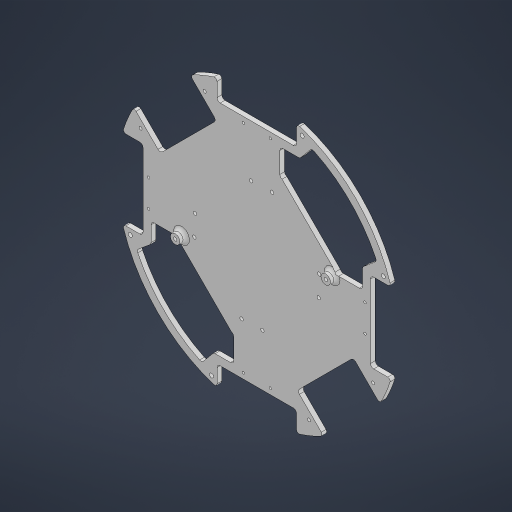
# Autodesk Inventor part: SecondPlate
Saved by Autodesk Inventor 2024.2 (Build 282272000, 272)
## iProperties
Created: 2023-12-22
Part Number: SecondPlate
Material: 一般
Document SubType Name: Modeling
Designer: Hanaoka
Density: 1 g/cm^3
Appearance: 既定
Author: Hanaoka
Autodesk Inventor part; units mm, degrees
(part 1 of 2)
ref_plane "YZ Plane" through (0, 0, 0) normal (1, 0, 0) x (0, 1, 0)
ref_plane "XZ Plane" through (0, 0, 0) normal (0, 1, 0) x (-1, 0, 0)
ref_plane "XY Plane" through (0, 0, 0) normal (0, 0, 1) x (1, 0, 0)
sketch "スケッチ1" plane through (0, 0, 0) normal (0, 0, 1) x (1, 0, 0)
  arc A0 (4.2199, -1.5405) -> (-52.5892, 55.2686) centre (-79.5487, -28.5) ccw projected
  arc A1 (2.792, -3.5) -> (4.2199, -1.5405) centre (2.792, -2) ccw projected
  line L0 (-6.0487, -3.5) -> (2.792, -3.5) projected
  circle A2 centre (0, 0) radius 2.5 projected
  circle A3 centre (0, 0) radius 1.3 projected
  arc A4 (-6.0487, -3.5) -> (-8.0487, -5.5) centre (-6.0487, -5.5) ccw projected
  line L1 (-8.0487, -51.5) -> (-8.0487, -5.5) projected
  arc A5 (-8.0487, -51.5) -> (-6.0487, -53.5) centre (-6.0487, -51.5) ccw projected
  line L2 (2.792, -53.5) -> (-6.0487, -53.5) projected
  arc A6 (4.2199, -55.4595) -> (2.792, -53.5) centre (2.792, -55) ccw projected
  arc A7 (-1.2521, -68.6701) -> (4.2199, -55.4595) centre (-79.5487, -28.5) ccw projected
  arc A8 (-3.6474, -69.046) -> (-1.2521, -68.6701) centre (-2.5867, -67.9854) ccw projected
  line L3 (-9.6341, -63.0593) -> (-3.6474, -69.046) projected
  arc A9 (-9.6341, -63.0593) -> (-13.8768, -63.0593) centre (-11.7555, -65.1806) ccw projected
  line L4 (-15.892, -65.0745) -> (-13.8768, -63.0593) projected
  line L5 (-39.4387, -88.6212) -> (-19.4276, -68.61) projected
  line L6 (-44.9895, -94.172) -> (-42.9742, -92.1567) projected
  arc A10 (-44.9895, -94.172) -> (-44.9895, -98.4146) centre (-42.8682, -96.2933) ccw projected
  line L7 (-39.0027, -104.4014) -> (-44.9895, -98.4146) projected
  arc A11 (-39.3786, -106.7966) -> (-39.0027, -104.4014) centre (-40.0634, -105.462) ccw projected
  arc A12 (-52.5892, -112.2686) -> (-39.3786, -106.7966) centre (-79.5487, -28.5) ccw projected
  arc A13 (-54.5487, -110.8408) -> (-52.5892, -112.2686) centre (-53.0487, -110.8408) ccw projected
  line L8 (-54.5487, -102) -> (-54.5487, -110.8408) projected
  arc A14 (-54.5487, -102) -> (-56.5487, -100) centre (-56.5487, -102) ccw projected
  line L9 (-102.5487, -100) -> (-56.5487, -100) projected
  arc A15 (-102.5487, -100) -> (-104.5487, -102) centre (-102.5487, -102) ccw projected
  line L10 (-104.5487, -110.8408) -> (-104.5487, -102) projected
  arc A16 (-106.5083, -112.2686) -> (-104.5487, -110.8408) centre (-106.0487, -110.8408) ccw projected
  arc A17 (-163.3174, -55.4595) -> (-106.5083, -112.2686) centre (-79.5487, -28.5) ccw projected
  circle A18 centre (-108.0487, -108.0487) radius 2.5 projected
  circle A19 centre (-108.0487, -108.0487) radius 1.3 projected
  arc A20 (-161.8895, -53.5) -> (-163.3174, -55.4595) centre (-161.8895, -55) ccw projected
  line L11 (-153.0487, -53.5) -> (-161.8895, -53.5) projected
  circle A21 centre (-159.0975, -57) radius 1.3 projected
  circle A22 centre (-159.0975, -57) radius 2.5 projected
  arc A23 (-153.0487, -53.5) -> (-151.0487, -51.5) centre (-153.0487, -51.5) ccw projected
  line L12 (-151.0487, -5.5) -> (-151.0487, -51.5) projected
  line L13 (-161.8895, -3.5) -> (-153.0487, -3.5) projected
  arc A24 (-151.0487, -5.5) -> (-153.0487, -3.5) centre (-153.0487, -5.5) ccw projected
  arc A25 (-163.3174, -1.5405) -> (-161.8895, -3.5) centre (-161.8895, -2) ccw projected
  arc A26 (-157.8454, 11.6701) -> (-163.3174, -1.5405) centre (-79.5487, -28.5) ccw projected
  arc A27 (-155.4501, 12.046) -> (-157.8454, 11.6701) centre (-156.5108, 10.9854) ccw projected
  line L14 (-149.4633, 6.0593) -> (-155.4501, 12.046) projected
  arc A28 (-149.4633, 6.0593) -> (-145.2207, 6.0593) centre (-147.342, 8.1806) ccw projected
  line L15 (-143.2054, 8.0745) -> (-145.2207, 6.0593) projected
  line L16 (-119.6588, 31.6212) -> (-139.6699, 11.61) projected
  line L17 (-114.108, 37.172) -> (-116.1232, 35.1567) projected
  arc A29 (-114.108, 37.172) -> (-114.108, 41.4146) centre (-116.2293, 39.2933) ccw projected
  line L18 (-120.0948, 47.4014) -> (-114.108, 41.4146) projected
  arc A30 (-119.7188, 49.7966) -> (-120.0948, 47.4014) centre (-119.0341, 48.462) ccw projected
  arc A31 (-106.5083, 55.2686) -> (-119.7188, 49.7966) centre (-79.5487, -28.5) ccw projected
  arc A32 (-104.5487, 53.8408) -> (-106.5083, 55.2686) centre (-106.0487, 53.8408) ccw projected
  line L19 (-104.5487, 45) -> (-104.5487, 53.8408) projected
  arc A33 (-104.5487, 45) -> (-102.5487, 43) centre (-102.5487, 45) ccw projected
  line L20 (-56.5487, 43) -> (-102.5487, 43) projected
  arc A34 (-52.5892, 55.2686) -> (-54.5487, 53.8408) centre (-53.0487, 53.8408) ccw projected
  line L21 (-54.5487, 53.8408) -> (-54.5487, 45) projected
  arc A35 (-56.5487, 43) -> (-54.5487, 45) centre (-56.5487, 45) ccw projected
  circle A36 centre (-51.0487, 51.0487) radius 2.5 projected
  circle A37 centre (-51.0487, 51.0487) radius 1.3 projected
  circle A38 centre (-11.5487, -37) radius 0.8 projected
  circle A39 centre (-11.5487, -20) radius 0.8 projected
  line L22 (-9.5487, -39.5) -> (-9.5487, -17.5) projected
  line L23 (-9.5487, -17.5) -> (-13.5487, -17.5) projected
  line L24 (-13.5487, -39.5) -> (-13.5487, -17.5) projected
  line L25 (-9.5487, -39.5) -> (-13.5487, -39.5) projected
  circle A40 centre (-71.0487, 39.5) radius 0.8 projected
  circle A41 centre (-88.0487, 39.5) radius 0.8 projected
  line L26 (-68.5487, 41.5) -> (-90.5487, 41.5) projected
  line L27 (-90.5487, 41.5) -> (-90.5487, 37.5) projected
  line L28 (-68.5487, 37.5) -> (-90.5487, 37.5) projected
  line L29 (-68.5487, 41.5) -> (-68.5487, 37.5) projected
  circle A42 centre (-147.5487, -20) radius 0.8 projected
  circle A43 centre (-147.5487, -37) radius 0.8 projected
  line L30 (-149.5487, -17.5) -> (-149.5487, -39.5) projected
  line L31 (-149.5487, -39.5) -> (-145.5487, -39.5) projected
  line L32 (-145.5487, -17.5) -> (-145.5487, -39.5) projected
  line L33 (-149.5487, -17.5) -> (-145.5487, -17.5) projected
  circle A44 centre (-88.0487, -96.5) radius 0.8 projected
  circle A45 centre (-71.0487, -96.5) radius 0.8 projected
  line L34 (-90.5487, -98.5) -> (-68.5487, -98.5) projected
  line L35 (-68.5487, -98.5) -> (-68.5487, -94.5) projected
  line L36 (-90.5487, -94.5) -> (-68.5487, -94.5) projected
  line L37 (-90.5487, -98.5) -> (-90.5487, -94.5) projected
  line L38 (-116.1232, 35.1567) -> (-119.6588, 31.6212)
  line L39 (-139.6699, 11.61) -> (-143.2054, 8.0745)
  line L40 (-15.892, -65.0745) -> (-19.4276, -68.61)
  line L41 (-42.9742, -92.1567) -> (-42.4775, -91.66)
  line L42 (-42.4775, -91.66) -> (-39.4387, -88.6212)
  line L43 (-49.5487, 45.911) -> (-49.5487, 38)
  line L44 (-51.5487, 36) -> (-72.0251, 36)
  line L45 (-73.4393, 35.4142) -> (-143.4629, -34.6094)
  line L46 (-5.1377, 1.5) -> (-13.0487, 1.5)
  line L47 (-15.0487, -0.5) -> (-15.0487, -20.9764)
  line L48 (-15.6345, -22.3906) -> (-85.6581, -92.4142)
  arc A46 (-3.3004, 4.2901) -> (-46.7586, 47.7483) centre (-79.5487, -28.5) ccw
  arc A47 (-5.1377, 1.5) -> (-3.3004, 4.2901) centre (-5.1377, 3.5) ccw
  arc A48 (-46.7586, 47.7483) -> (-49.5487, 45.911) centre (-47.5487, 45.911) ccw
  arc A49 (-51.5487, 36) -> (-49.5487, 38) centre (-51.5487, 38) ccw
  arc A50 (-13.0487, 1.5) -> (-15.0487, -0.5) centre (-13.0487, -0.5) ccw
  arc A51 (-15.6345, -22.3906) -> (-15.0487, -20.9764) centre (-17.0487, -20.9764) ccw
  arc A52 (-72.0251, 36) -> (-73.4393, 35.4142) centre (-72.0251, 34) ccw
  line L49 (-129.6643, 21.6156) -> (-29.4331, -78.6156) construction
  line L50 (-153.9597, -58.5) -> (-146.0487, -58.5)
  line L51 (-144.0487, -56.5) -> (-144.0487, -36.0236)
  line L52 (-109.5487, -102.911) -> (-109.5487, -95)
  line L53 (-107.5487, -93) -> (-87.0724, -93)
  arc A53 (-155.7971, -61.2901) -> (-112.3389, -104.7483) centre (-79.5487, -28.5) ccw
  arc A54 (-112.3389, -104.7483) -> (-109.5487, -102.911) centre (-111.5487, -102.911) ccw
  arc A55 (-153.9597, -58.5) -> (-155.7971, -61.2901) centre (-153.9597, -60.5) ccw
  arc A56 (-146.0487, -58.5) -> (-144.0487, -56.5) centre (-146.0487, -56.5) ccw
  arc A57 (-107.5487, -93) -> (-109.5487, -95) centre (-107.5487, -95) ccw
  arc A58 (-87.0724, -93) -> (-85.6581, -92.4142) centre (-87.0724, -91) ccw
  arc A59 (-143.4629, -34.6094) -> (-144.0487, -36.0236) centre (-142.0487, -36.0236) ccw
  line L54 (-9.6341, -63.0593) -> (-36.5042, -36.1892)
  line L55 (-39.3326, -36.1892) -> (-71.8595, -68.7161)
  line L56 (-71.8595, -71.5445) -> (-44.9895, -98.4146)
  arc A60 (-36.5042, -36.1892) -> (-39.3326, -36.1892) centre (-37.9184, -37.6034) ccw
  arc A61 (-71.8595, -68.7161) -> (-71.8595, -71.5445) centre (-70.4453, -70.1303) ccw
  line L57 (-114.108, 41.4146) -> (-87.2379, 14.5445)
  line L58 (-87.2379, 11.7161) -> (-119.7648, -20.8108)
  line L59 (-122.5933, -20.8108) -> (-149.4633, 6.0593)
  arc A62 (-87.2379, 11.7161) -> (-87.2379, 14.5445) centre (-88.6521, 13.1303) ccw
  arc A63 (-122.5933, -20.8108) -> (-119.7648, -20.8108) centre (-121.179, -19.3966) ccw
  arc A64 (4.2199, -55.4595) -> (4.2199, -55.4595) centre (-79.5487, -28.5) ccw
  arc A65 (-52.5892, -112.2686) -> (-52.5892, -112.2686) centre (-79.5487, -28.5) ccw
  arc A66 (-54.5487, -102) -> (-56.5487, -100) centre (-56.5487, -102) ccw
  point P0 (0, 0)
  point P1 (-49.5487, 48.8886)
  point P2 (-2.1601, 1.5)
  point P3 (-2.1601, 1.5)
  point P4 (-49.5487, 48.8886)
  point P5 (-73.2737, -70.1303)
  point P6 (-52.5892, -112.2686)
  dimension "d2" = 5
  dimension "d3" = 2
  dimension "d4" = 5
  dimension "d5" = 5
  dimension "d6" = 1.5
  dimension "d7" = 1.5
  dimension "d8" = 30
  dimension "d9" = 30
  dimension "d12" = 40
  dimension "d13" = 2
  constraints: 47 point on circle, 44 end point, 21 centre point, 20 tangent, 19 symmetric about line, 11 parallel, 8 equal radius, 8 point on line, 4 collinear, 3 coincident, 2 midpoint, 1 perpendicular, 8 other
  measures "d2" radial gap between concentric circles of A0 A46
  measures "d3" radius of A47
  measures "d4" distance between parallel lines of L0 L46
  measures "d5" distance between parallel lines of L21 L43
  measures "d6" distance between parallel lines of L44 L28
  measures "d7" distance between parallel lines of L47 L24
  measures "d8" distance between parallel lines of L16 L45
  measures "d9" distance between parallel lines of L5 L48
  measures "d12" distance of point (-73.274, -70.13) L7.end
  measures "d13" radius of A60
extrude "押し出し1" add sketch "スケッチ1" along normal blind 1 contours A1 L0 A4 L1 A5 L2 A6 A7 A8 L3 L54 L48 A51 L47 A50 L46 A47 A46 A48 L43 A49 L44 A52 L45 L57 L18 A30 A31 A32 L19 A33 L20 A35 L21 A34 A0 | A27 L14 L59 L45 A59 L51 A56 L50 A55 A53 A54 L52 A57 L53 A58 L48 L56 L7 A11 A12 A13 L8 A14 L9 A15 L10 A16 A17 A20 L11 A23 L12 A24 L13 A25 A26 | L57 A62 L58 A63 L59 L45 | L45 A52 L44 A49 L43 A48 A46 A47 L46 A50 L47 A51 L48 L54 A60 L55 A61 L56 A58 L53 A57 L52 A54 A53 A55 L50 A56 L51 A59 L59 A63 L58 A62 L57 | L48 L56 A61 L55 A60 L54 | A2 | A18 | A22 | A36 | L25 L24 L23 L22 | L29 L28 L27 L26 | L33 L32 L31 L30 | L37 L36 L35 L34
sketch "スケッチ2" plane through (0, 0, 0) normal (0, 0, -1) x (-1, 0, 0)
  arc A0 (-4.2199, -1.5405) -> (-2.792, -3.5) centre (-2.792, -2) ccw projected
  line L0 (6.0487, -3.5) -> (-2.792, -3.5) projected
  arc A1 (8.0487, -5.5) -> (6.0487, -3.5) centre (6.0487, -5.5) ccw projected
  line L1 (8.0487, -51.5) -> (8.0487, -5.5) projected
  arc A2 (6.0487, -53.5) -> (8.0487, -51.5) centre (6.0487, -51.5) ccw projected
  line L2 (-2.792, -53.5) -> (6.0487, -53.5) projected
  arc A3 (-2.792, -53.5) -> (-4.2199, -55.4595) centre (-2.792, -55) ccw projected
  arc A4 (-4.2199, -55.4595) -> (1.2521, -68.6701) centre (79.5487, -28.5) ccw projected
  arc A5 (1.2521, -68.6701) -> (3.6474, -69.046) centre (2.5867, -67.9854) ccw projected
  line L3 (32.9687, -39.7247) -> (3.6474, -69.046) projected
  line L4 (39.0027, -104.4014) -> (68.324, -75.0801) projected
  arc A6 (39.0027, -104.4014) -> (39.3786, -106.7966) centre (40.0634, -105.462) ccw projected
  arc A7 (39.3786, -106.7966) -> (52.5892, -112.2686) centre (79.5487, -28.5) ccw projected
  arc A8 (52.5892, -112.2686) -> (54.5487, -110.8408) centre (53.0487, -110.8408) ccw projected
  line L5 (54.5487, -102) -> (54.5487, -110.8408) projected
  arc A9 (56.5487, -100) -> (54.5487, -102) centre (56.5487, -102) ccw projected
  line L6 (102.5487, -100) -> (56.5487, -100) projected
  arc A10 (104.5487, -102) -> (102.5487, -100) centre (102.5487, -102) ccw projected
  line L7 (104.5487, -110.8408) -> (104.5487, -102) projected
  arc A11 (104.5487, -110.8408) -> (106.5083, -112.2686) centre (106.0487, -110.8408) ccw projected
  arc A12 (106.5083, -112.2686) -> (163.3174, -55.4595) centre (79.5487, -28.5) ccw projected
  arc A13 (163.3174, -55.4595) -> (161.8895, -53.5) centre (161.8895, -55) ccw projected
  line L8 (153.0487, -53.5) -> (161.8895, -53.5) projected
  arc A14 (151.0487, -51.5) -> (153.0487, -53.5) centre (153.0487, -51.5) ccw projected
  line L9 (151.0487, -5.5) -> (151.0487, -51.5) projected
  arc A15 (153.0487, -3.5) -> (151.0487, -5.5) centre (153.0487, -5.5) ccw projected
  line L10 (161.8895, -3.5) -> (153.0487, -3.5) projected
  arc A16 (161.8895, -3.5) -> (163.3174, -1.5405) centre (161.8895, -2) ccw projected
  arc A17 (163.3174, -1.5405) -> (157.8454, 11.6701) centre (79.5487, -28.5) ccw projected
  arc A18 (157.8454, 11.6701) -> (155.4501, 12.046) centre (156.5108, 10.9854) ccw projected
  line L11 (126.1288, -17.2753) -> (155.4501, 12.046) projected
  line L12 (120.0948, 47.4014) -> (90.7735, 18.0801) projected
  arc A19 (120.0948, 47.4014) -> (119.7188, 49.7966) centre (119.0341, 48.462) ccw projected
  arc A20 (119.7188, 49.7966) -> (106.5083, 55.2686) centre (79.5487, -28.5) ccw projected
  arc A21 (106.5083, 55.2686) -> (104.5487, 53.8408) centre (106.0487, 53.8408) ccw projected
  line L13 (104.5487, 45) -> (104.5487, 53.8408) projected
  arc A22 (102.5487, 43) -> (104.5487, 45) centre (102.5487, 45) ccw projected
  line L14 (56.5487, 43) -> (102.5487, 43) projected
  arc A23 (54.5487, 45) -> (56.5487, 43) centre (56.5487, 45) ccw projected
  line L15 (54.5487, 53.8408) -> (54.5487, 45) projected
  arc A24 (54.5487, 53.8408) -> (52.5892, 55.2686) centre (53.0487, 53.8408) ccw projected
  arc A25 (52.5892, 55.2686) -> (-4.2199, -1.5405) centre (79.5487, -28.5) ccw projected
  line L16 (68.5487, 37.5) -> (90.5487, 37.5) projected
  line L17 (68.5487, 41.5) -> (90.5487, 41.5) projected
  line L18 (90.5487, 41.5) -> (90.5487, 37.5) projected
  line L19 (68.5487, 41.5) -> (68.5487, 37.5) projected
  line L20 (149.5487, -17.5) -> (149.5487, -39.5) projected
  line L21 (149.5487, -17.5) -> (145.5487, -17.5) projected
  line L22 (145.5487, -17.5) -> (145.5487, -39.5) projected
  line L23 (149.5487, -39.5) -> (145.5487, -39.5) projected
  line L24 (90.5487, -98.5) -> (68.5487, -98.5) projected
  line L25 (90.5487, -94.5) -> (68.5487, -94.5) projected
  line L26 (90.5487, -98.5) -> (90.5487, -94.5) projected
  line L27 (68.5487, -98.5) -> (68.5487, -94.5) projected
  line L28 (13.5487, -39.5) -> (13.5487, -17.5) projected
  line L29 (9.5487, -17.5) -> (13.5487, -17.5) projected
  line L30 (9.5487, -39.5) -> (9.5487, -17.5) projected
  line L31 (9.5487, -39.5) -> (13.5487, -39.5) projected
  circle A26 centre (51.0487, 51.0487) radius 2.5
  circle A27 centre (0, 0) radius 2.5
  circle A28 centre (159.0975, -57) radius 2.5
  circle A29 centre (108.0487, -108.0487) radius 2.5
  line L32 (17.3233, 33.7254) -> (141.7741, -90.7254) construction
  circle A30 centre (118.7932, -38.0459) radius 1.1
  circle A31 centre (89.0947, -67.7444) radius 1.1
  line L33 (118.7932, -38.0459) -> (89.0947, -67.7444) construction
  line L34 (114.108, 6.0593) -> (44.9895, -63.0593) construction
  circle A32 centre (70.0028, 10.7444) radius 1.1
  circle A33 centre (40.3043, -18.9541) radius 1.1
  line L35 (70.0028, 10.7444) -> (40.3043, -18.9541) construction
  line L36 (149.5487, -17.5) -> (149.1952, -17.8536) construction
  arc A34 (149.5487, -18.2071) -> (148.8416, -17.5) centre (149.1952, -17.8536) ccw
  line L37 (149.1952, -17.5) -> (149.1952, -17.8536) construction
  line L38 (149.1952, -17.8536) -> (149.5487, -17.8536) construction
  line L39 (145.5487, -17.5) -> (145.9023, -17.8536) construction
  line L40 (149.5487, -39.5) -> (149.1952, -39.1464) construction
  line L41 (145.5487, -39.5) -> (145.9023, -39.1464) construction
  line L42 (145.9023, -17.8536) -> (145.9023, -17.5) construction
  line L43 (145.9023, -17.8536) -> (145.5487, -17.8536) construction
  line L44 (149.1952, -39.1464) -> (149.5487, -39.1464) construction
  line L45 (145.9023, -39.1464) -> (145.5487, -39.1464) construction
  line L46 (145.9023, -39.1464) -> (145.9023, -39.5) construction
  line L47 (149.1952, -39.1464) -> (149.1952, -39.5) construction
  arc A35 (146.2558, -17.5) -> (145.5487, -18.2071) centre (145.9023, -17.8536) ccw
  arc A36 (148.8416, -39.5) -> (149.5487, -38.7929) centre (149.1952, -39.1464) ccw
  arc A37 (145.5487, -38.7929) -> (146.2558, -39.5) centre (145.9023, -39.1464) ccw
  arc A38 (69.2558, 41.5) -> (68.5487, 40.7929) centre (68.9023, 41.1464) ccw
  arc A39 (68.5487, 38.2071) -> (69.2558, 37.5) centre (68.9023, 37.8536) ccw
  arc A40 (90.5487, 40.7929) -> (89.8416, 41.5) centre (90.1952, 41.1464) ccw
  arc A41 (89.8416, 37.5) -> (90.5487, 38.2071) centre (90.1952, 37.8536) ccw
  arc A42 (9.5487, -38.7929) -> (10.2558, -39.5) centre (9.9023, -39.1464) ccw
  arc A43 (12.8416, -39.5) -> (13.5487, -38.7929) centre (13.1952, -39.1464) ccw
  arc A44 (10.2558, -17.5) -> (9.5487, -18.2071) centre (9.9023, -17.8536) ccw
  arc A45 (13.5487, -18.2071) -> (12.8416, -17.5) centre (13.1952, -17.8536) ccw
  arc A46 (89.8416, -98.5) -> (90.5487, -97.7929) centre (90.1952, -98.1464) ccw
  arc A47 (90.5487, -95.2071) -> (89.8416, -94.5) centre (90.1952, -94.8536) ccw
  arc A48 (68.5487, -97.7929) -> (69.2558, -98.5) centre (68.9023, -98.1464) ccw
  arc A49 (69.2558, -94.5) -> (68.5487, -95.2071) centre (68.9023, -94.8536) ccw
  line L48 (68.324, -75.0801) -> (32.9687, -39.7247) projected
  line L49 (90.7735, 18.0801) -> (126.1288, -17.2753) projected
  circle A50 centre (88.0487, 39.5) radius 0.8 projected
  circle A51 centre (71.0487, 39.5) radius 0.8 projected
  circle A52 centre (147.5487, -20) radius 0.8 projected
  circle A53 centre (147.5487, -37) radius 0.8 projected
  circle A54 centre (88.0487, -96.5) radius 0.8 projected
  circle A55 centre (71.0487, -96.5) radius 0.8 projected
  circle A56 centre (11.5487, -20) radius 0.8 projected
  circle A57 centre (11.5487, -37) radius 0.8 projected
  circle A58 centre (0, 0) radius 1.3 projected
  circle A59 centre (51.0487, 51.0487) radius 1.3 projected
  circle A60 centre (159.0975, -57) radius 1.3 projected
  circle A61 centre (108.0487, -108.0487) radius 1.3 projected
  point P0 (0, 0)
  point P1 (103.9439, -52.8952)
  point P2 (79.5487, -28.5)
  point P3 (68.5487, 41.5)
  point P4 (9.5487, -39.5)
  point P5 (90.5487, -98.5)
  point P6 (69.2558, 37.5)
  point P7 (13.5487, -38.7929)
  point P8 (68.5487, -95.2071)
  point P9 (69.2558, -94.5)
  point P10 (89.8416, -94.5)
  point P11 (90.5487, -97.7929)
  point P12 (89.8416, -98.5)
  point P13 (69.2558, -98.5)
  dimension "d16" = 5
  dimension "d17" = 2.2
  dimension "d18" = 42
  dimension "d19" = 34.5
  dimension "d20" = 34.5
  dimension "d61" = 0.5
  dimension "d65" = 360
  constraints: 38 point on circle, 32 end point, 24 centre point, 17 point on line, 8 equal length, 8 equal radius, 4 coincident, 4 perpendicular, 3 parallel, 2 midpoint, 1 vertical, 71 other
  measures "d16" diameter of A26
  measures "d17" diameter of A31
  measures "d18" distance of L33.start L33.end
  measures "d19" distance of point (103.944, -52.895) point (79.549, -28.5)
  measures "d20" distance between parallel lines of L34 L35
  measures "d61" distance of L20.start L36.end
extrude "押し出し2" add sketch "スケッチ2" along normal blind 2 contours A25 A24 L15 A23 L14 A22 L13 A21 A20 A19 L12 L49 L11 A18 A17 A16 L10 A15 L9 A14 L8 A13 A12 A11 L7 A10 L6 A9 L5 A8 A7 A6 L4 L48 L3 A5 A4 A3 L2 A2 L1 A1 L0 A0 | L19 L17 L18 L16 | A39 L19 | L16 A39 | L16 A41 | A38 L19 | L18 A41 | A38 L17 | L18 A40 | A40 L17 | A34 L20 | L20 L23 L22 L21 | L21 A34 | A36 L20 | L21 A35 | A36 L23 | L22 A35 | A37 L23 | L22 A37 | A46 L24 | L24 L27 L25 L26 | L26 A46 | A48 L24 | L26 A47 | A48 L27 | L25 A47 | A49 L27 | L25 A49 | L31 L30 L29 L28 | A43 L31 | L28 A43 | L28 A45 | A42 L31 | L29 A45 | A42 L30 | L29 A44 | A44 L30 | A26 | A27 | A28 | A29 | A30 | A31 | A32 | A33
extrude "押し出し3" cut sketch "スケッチ2" along normal mid plane 5 contours A30 | A31 | A32 | A33
sketch "スケッチ3" plane through (0, 0, 1) normal (0, 0, 1) x (1, 0, 0)
  circle A0 centre (-40.6579, -32.0355) radius 1.1
  circle A1 centre (-76.0132, -67.3909) radius 1.1
  circle A2 centre (-83.0843, 10.3909) radius 1.1
  circle A3 centre (-118.4396, -24.9645) radius 1.1
  line L0 (-83.0843, 10.3909) -> (-40.6579, -32.0355) construction
  line L1 (-40.6579, -32.0355) -> (-76.0132, -67.3909) construction
  line L2 (-76.0132, -67.3909) -> (-118.4396, -24.9645) construction
  line L3 (-118.4396, -24.9645) -> (-83.0843, 10.3909) construction
  line L4 (-17.3233, 33.7254) -> (-141.7741, -90.7254) construction
  arc A4 (4.2199, -1.5405) -> (-52.5892, 55.2686) centre (-79.5487, -28.5) ccw projected
  arc A5 (-163.3174, -55.4595) -> (-106.5083, -112.2686) centre (-79.5487, -28.5) ccw projected
  line L5 (-97.8445, 22.3227) -> (-130.3714, -10.2042) projected
  line L6 (-114.108, 6.0593) -> (-44.9895, -63.0593) construction
  line L7 (-61.2529, -79.3227) -> (-28.726, -46.7958) projected
  circle A6 centre (-40.6579, -32.0355) radius 2.5
  circle A7 centre (-76.0132, -67.3909) radius 2.5
  circle A8 centre (-118.4396, -24.9645) radius 2.5
  circle A9 centre (-83.0843, 10.3909) radius 2.5
  point P0 (0, 0)
  point P1 (-58.3355, -49.7132)
  point P2 (-97.2264, -46.1777)
  dimension "d23" = 2.2
  dimension "d24" = 50
  dimension "d25" = 60
  dimension "d26" = 5
  constraints: 12 end point, 8 centre point, 6 equal radius, 4 coincident, 4 midpoint, 4 parallel, 2 point on circle, 2 point on line
  measures "d23" diameter of A1
  measures "d24" distance of L0.end L1.end
  measures "d25" distance of L0.start L0.end
  measures "d26" diameter of A7
extrude "押し出し4" cut sketch "スケッチ3" against normal up to surface (3 mm away) contours A0 | A1 | A2 | A3
sketch "スケッチ5" plane through (0, 0, 1) normal (0, 0, 1) x (1, 0, 0)
  arc A0 (-25.87, 37.9067) -> (-25.9576, 39.3987) centre (-26.5771, 38.6138) ccw projected
  arc A1 (-25.9576, 39.3987) -> (-45.1385, 50.8611) centre (-79.5487, -28.5) ccw projected
  arc A2 (-45.1385, 50.8611) -> (-47.4757, 50.3004) centre (-45.9341, 49.0262) ccw projected
  line L0 (-47.4757, 50.3004) -> (-53.7364, 42.7258) projected
  arc A3 (-55.278, 42) -> (-53.7364, 42.7258) centre (-55.278, 44) ccw projected
  line L1 (-55.278, 42) -> (-63.0487, 42) projected
  arc A4 (-63.0487, 42) -> (-65.0487, 40) centre (-63.0487, 40) ccw projected
  line L2 (-65.0487, 40) -> (-65.0487, 27.1035) projected
  arc A5 (-65.0487, 27.1035) -> (-63.6177, 25.1861) centre (-63.0487, 27.1035) ccw projected
  arc A6 (-25.8626, -12.569) -> (-63.6177, 25.1861) centre (-79.5487, -28.5) ccw projected
  arc A7 (-25.8626, -12.569) -> (-23.9452, -14) centre (-23.9452, -12) ccw projected
  line L3 (-23.9452, -14) -> (-11.0487, -14) projected
  arc A8 (-11.0487, -14) -> (-9.0487, -12) centre (-11.0487, -12) ccw projected
  line L4 (-9.0487, -12) -> (-9.0487, -4.2293) projected
  arc A9 (-8.3229, -2.6877) -> (-9.0487, -4.2293) centre (-7.0487, -4.2293) ccw projected
  line L5 (-8.3229, -2.6877) -> (-0.7484, 3.573) projected
  arc A10 (-0.7484, 3.573) -> (-0.1876, 5.9102) centre (-2.0226, 5.1146) ccw projected
  arc A11 (-0.1876, 5.9102) -> (-11.65, 25.0912) centre (-79.5487, -28.5) ccw projected
  arc A12 (-11.65, 25.0912) -> (-13.1421, 25.1787) centre (-12.435, 24.4716) ccw projected
  line L6 (-13.1421, 25.1787) -> (-17.3018, 21.0191) projected
  arc A13 (-18.716, 21.0191) -> (-17.3018, 21.0191) centre (-18.0089, 21.7262) ccw projected
  line L7 (-18.716, 21.0191) -> (-30.0297, 32.3328) projected
  arc A14 (-30.0297, 33.747) -> (-30.0297, 32.3328) centre (-29.3226, 33.0399) ccw projected
  line L8 (-30.0297, 33.747) -> (-25.87, 37.9067) projected
  circle A15 centre (-45.9341, 49.0262) radius 1 projected
  circle A16 centre (-2.0226, 5.1146) radius 1 projected
  circle A17 centre (-63.0487, 35.9205) radius 1 projected
  circle A18 centre (-15.1282, -12) radius 1 projected
  arc A19 (-4.7333, 7.4395) -> (-43.6092, 46.3155) centre (-79.5487, -28.5) ccw
  arc A20 (4.2199, -1.5405) -> (-52.5892, 55.2686) centre (-79.5487, -28.5) ccw projected
  line L9 (-5.2619, 5.0319) -> (-12.3229, -0.8044)
  line L10 (-13.0487, -2.346) -> (-13.0487, -12)
  line L11 (-15.0487, -14) -> (-23.9452, -14)
  arc A21 (-25.8626, -12.569) -> (-63.6177, 25.1861) centre (-79.5487, -28.5) ccw
  line L12 (-17.3233, 33.7254) -> (-39.9507, 11.098) construction
  line L13 (-46.0168, 45.7869) -> (-51.8531, 38.7258)
  line L14 (-53.3947, 38) -> (-63.0487, 38)
  line L15 (-65.0487, 36) -> (-65.0487, 27.1035)
  arc A22 (-5.2619, 5.0319) -> (-4.7333, 7.4395) centre (-6.5361, 6.5735) ccw
  arc A23 (-12.3229, -0.8044) -> (-13.0487, -2.346) centre (-11.0487, -2.346) ccw
  arc A24 (-15.0487, -14) -> (-13.0487, -12) centre (-15.0487, -12) ccw
  arc A25 (-25.8626, -12.569) -> (-23.9452, -14) centre (-23.9452, -12) ccw
  arc A26 (-65.0487, 27.1035) -> (-63.6177, 25.1861) centre (-63.0487, 27.1035) ccw
  arc A27 (-63.0487, 38) -> (-65.0487, 36) centre (-63.0487, 36) ccw
  arc A28 (-53.3947, 38) -> (-51.8531, 38.7258) centre (-53.3947, 40) ccw
  arc A29 (-43.6092, 46.3155) -> (-46.0168, 45.7869) centre (-44.4752, 44.5127) ccw
  line L16 (-97.8445, 22.3227) -> (-130.3714, -10.2042) projected
  line L17 (-114.108, 6.0593) -> (-44.9895, -63.0593) construction
  line L18 (-61.2529, -79.3227) -> (-28.726, -46.7958) projected
  arc A30 (-133.2349, -44.431) -> (-135.1522, -43) centre (-135.1522, -45) ccw
  arc A31 (-133.2349, -44.431) -> (-95.4798, -82.1861) centre (-79.5487, -28.5) ccw
  arc A32 (-154.3642, -64.4395) -> (-115.4882, -103.3155) centre (-79.5487, -28.5) ccw
  line L19 (-113.0806, -102.7869) -> (-107.2443, -95.7258)
  line L20 (-105.7028, -95) -> (-96.0487, -95)
  line L21 (-94.0487, -93) -> (-94.0487, -84.1035)
  line L22 (-153.8356, -62.0319) -> (-146.7745, -56.1956)
  line L23 (-146.0487, -54.654) -> (-146.0487, -45)
  line L24 (-144.0487, -43) -> (-135.1522, -43)
  arc A33 (-115.4882, -103.3155) -> (-113.0806, -102.7869) centre (-114.6222, -101.5127) ccw
  arc A34 (-105.7028, -95) -> (-107.2443, -95.7258) centre (-105.7028, -97) ccw
  arc A35 (-96.0487, -95) -> (-94.0487, -93) centre (-96.0487, -93) ccw
  arc A36 (-94.0487, -84.1035) -> (-95.4798, -82.1861) centre (-96.0487, -84.1035) ccw
  arc A37 (-144.0487, -43) -> (-146.0487, -45) centre (-144.0487, -45) ccw
  arc A38 (-146.7745, -56.1956) -> (-146.0487, -54.654) centre (-148.0487, -54.654) ccw
  arc A39 (-153.8356, -62.0319) -> (-154.3642, -64.4395) centre (-152.5614, -63.5735) ccw
  line L25 (-46.0168, 45.7869) -> (-41.7384, 50.9631)
  line L26 (-5.2619, 5.0319) -> (-0.0857, 9.3103)
  line L27 (-65.0487, 36) -> (-65.0487, 43)
  line L28 (-15.0487, -14) -> (-8.0487, -14)
  line L29 (-56.5487, 43) -> (-102.5487, 43) projected
  line L30 (-8.0487, -51.5) -> (-8.0487, -5.5) projected
  arc A40 (-6.0487, -3.5) -> (-8.0487, -5.5) centre (-6.0487, -5.5) ccw projected
  line L31 (-6.0487, -3.5) -> (2.792, -3.5) projected
  arc A41 (2.792, -3.5) -> (4.2199, -1.5405) centre (2.792, -2) ccw projected
  line L32 (-54.5487, 53.8408) -> (-54.5487, 45) projected
  arc A42 (-56.5487, 43) -> (-54.5487, 45) centre (-56.5487, 45) ccw projected
  arc A43 (-52.5892, 55.2686) -> (-54.5487, 53.8408) centre (-53.0487, 53.8408) ccw projected
  arc A44 (-163.3174, -55.4595) -> (-106.5083, -112.2686) centre (-79.5487, -28.5) ccw
  line L33 (-144.0487, -43) -> (-151.0487, -43)
  line L34 (-94.0487, -93) -> (-94.0487, -100)
  line L35 (-56.5487, -100) -> (-102.5487, -100)
  arc A45 (-102.5487, -100) -> (-104.5487, -102) centre (-102.5487, -102) ccw
  line L36 (-104.5487, -102) -> (-104.5487, -110.8408)
  arc A46 (-106.5083, -112.2686) -> (-104.5487, -110.8408) centre (-106.0487, -110.8408) ccw
  line L37 (-161.8895, -53.5) -> (-153.0487, -53.5)
  arc A47 (-153.0487, -53.5) -> (-151.0487, -51.5) centre (-153.0487, -51.5) ccw
  arc A48 (-161.8895, -53.5) -> (-163.3174, -55.4595) centre (-161.8895, -55) ccw
  line L38 (-102.5487, -100) -> (-56.5487, -100) projected
  arc A49 (-102.5487, -100) -> (-104.5487, -102) centre (-102.5487, -102) ccw projected
  line L39 (-104.5487, -110.8408) -> (-104.5487, -102) projected
  arc A50 (-106.5083, -112.2686) -> (-104.5487, -110.8408) centre (-106.0487, -110.8408) ccw projected
  arc A51 (-163.3174, -55.4595) -> (-106.5083, -112.2686) centre (-79.5487, -28.5) ccw projected
  arc A52 (-161.8895, -53.5) -> (-163.3174, -55.4595) centre (-161.8895, -55) ccw projected
  line L40 (-153.0487, -53.5) -> (-161.8895, -53.5) projected
  arc A53 (-153.0487, -53.5) -> (-151.0487, -51.5) centre (-153.0487, -51.5) ccw projected
  line L41 (-151.0487, -5.5) -> (-151.0487, -51.5) projected
  arc A54 (-30.0357, -12.6111) -> (-63.6598, 21.0131) centre (-79.5487, -28.5) ccw
  line L42 (-65.0487, 22.9174) -> (-65.0487, 27.1035)
  line L43 (-28.1313, -14) -> (-23.9452, -14)
  arc A55 (-65.0487, 22.9174) -> (-63.6598, 21.0131) centre (-63.0487, 22.9174) ccw
  arc A56 (-30.0357, -12.6111) -> (-28.1313, -14) centre (-28.1313, -12) ccw
  arc A57 (-129.0618, -44.3889) -> (-95.4376, -78.0131) centre (-79.5487, -28.5) ccw
  line L44 (-130.9661, -43) -> (-135.1522, -43)
  line L45 (-94.0487, -79.9174) -> (-94.0487, -84.1035)
  arc A58 (-129.0618, -44.3889) -> (-130.9661, -43) centre (-130.9661, -45) ccw
  arc A59 (-94.0487, -79.9174) -> (-95.4376, -78.0131) centre (-96.0487, -79.9174) ccw
  point P0 (0, 0)
  point P1 (-4.0674, 6.0192)
  point P2 (-45.0296, 46.9813)
  point P3 (-13.0487, -1.4043)
  point P4 (-13.0487, -14)
  point P5 (-25.4585, -14)
  point P6 (-25.4585, -14)
  point P7 (-65.0487, 25.5902)
  point P8 (-45.0296, 46.9813)
  point P9 (-52.453, 38)
  point P10 (-65.0487, 38)
  point P11 (-65.0487, 25.5902)
  point P12 (-27.5689, 36.2078)
  point P13 (-63.6177, 25.1861)
  point P14 (-25.8626, -12.569)
  point P15 (-14.841, 23.4798)
  point P16 (-17.497, -14)
  point P17 (-95.4798, -82.1861)
  point P18 (-1.2786, 8.3243)
  point P19 (-42.7244, 49.7702)
  point P20 (-29.6113, -14)
  point P21 (-65.0487, 21.4375)
  point P22 (-94.0487, -84.1035)
  dimension "d38" = 5
  dimension "d39" = 4
  dimension "d41" = 4
  dimension "d42" = 2
  dimension "d43" = 2
  dimension "d52" = 52
  dimension "d53" = 2
  constraints: 73 point on circle, 54 end point, 53 symmetric about line, 31 centre point, 21 point on line, 20 tangent, 7 equal radius, 6 collinear, 3 coincident, 3 midpoint, 2 parallel, 2 perpendicular, 1 vertical, 18 other
  measures "d38" radial gap between concentric circles of A20 A19
  measures "d39" distance between parallel lines of L5 L9
  measures "d41" distance between parallel lines of L4 L10
  measures "d42" radius of A22
  measures "d43" radius of A29
  measures "d52" radius of A54
  measures "d53" radius of A55
extrude "押し出し6" cut sketch "スケッチ5" against normal up to surface (3 mm away) contours A19 L6 A13 L7 A14 L8 | L8 A14 L7 A13 L6 A19 A22 L9 A23 L10 A24 L3 A7 A6 A5 L2 A27 L14 A28 L13 A29 | A5 A6 A7 L43 A56 A54 A55 L42 | A17 | A18 | A31 A36 L21 A35 L20 A34 L19 A33 A32 A39 L22 A38 L23 A37 L24 A30 | A30 L44 A58 A57 A59 L45 A36 A31
sketch "ハンドル" plane through (0, 0, 1) normal (0, 0, 1) x (1, 0, 0)
  circle A0 centre (-118.4396, -24.9645) radius 1.1 projected
  circle A1 centre (-40.6579, -32.0355) radius 1.1 projected
  circle A2 centre (-76.0132, -67.3909) radius 1.1 projected
  circle A3 centre (-83.0843, 10.3909) radius 1.1 projected
  circle A4 centre (-89.0947, -67.7444) radius 1.1 projected
  circle A5 centre (-118.7932, -38.0459) radius 1.1 projected
  circle A6 centre (-40.3043, -18.9541) radius 1.1 projected
  circle A7 centre (-70.0028, 10.7444) radius 1.1 projected
  circle A8 centre (-79.5487, -28.5) radius 49 construction
  circle A9 centre (-32.2184, -15.8179) radius 1.1
  line L0 (-39.9507, 11.098) -> (-119.1467, -68.098) construction
  line L1 (-32.2184, -15.8179) -> (-126.8791, -41.1821) construction
  circle A10 centre (-126.8791, -41.1821) radius 1.1
  line L2 (-56.5487, 43) -> (-102.5487, 43) projected
  arc A11 (-104.5487, 45) -> (-102.5487, 43) centre (-102.5487, 45) ccw projected
  line L3 (-104.5487, 45) -> (-104.5487, 53.8408) projected
  arc A12 (-104.5487, 53.8408) -> (-106.5083, 55.2686) centre (-106.0487, 53.8408) ccw projected
  arc A13 (-106.5083, 55.2686) -> (-119.7188, 49.7966) centre (-79.5487, -28.5) ccw projected
  arc A14 (-119.7188, 49.7966) -> (-120.0948, 47.4014) centre (-119.0341, 48.462) ccw projected
  line L4 (-120.0948, 47.4014) -> (-90.7735, 18.0801) projected
  line L5 (-126.1288, -17.2753) -> (-155.4501, 12.046) projected
  arc A15 (-155.4501, 12.046) -> (-157.8454, 11.6701) centre (-156.5108, 10.9854) ccw projected
  arc A16 (-157.8454, 11.6701) -> (-163.3174, -1.5405) centre (-79.5487, -28.5) ccw projected
  arc A17 (-163.3174, -1.5405) -> (-161.8895, -3.5) centre (-161.8895, -2) ccw projected
  line L6 (-161.8895, -3.5) -> (-153.0487, -3.5) projected
  arc A18 (-151.0487, -5.5) -> (-153.0487, -3.5) centre (-153.0487, -5.5) ccw projected
  line L7 (-151.0487, -5.5) -> (-151.0487, -51.5) projected
  line L8 (-102.5487, -100) -> (-56.5487, -100) projected
  arc A19 (-54.5487, -102) -> (-56.5487, -100) centre (-56.5487, -102) ccw projected
  line L9 (-54.5487, -102) -> (-54.5487, -110.8408) projected
  arc A20 (-54.5487, -110.8408) -> (-52.5892, -112.2686) centre (-53.0487, -110.8408) ccw projected
  arc A21 (-52.5892, -112.2686) -> (-39.3786, -106.7966) centre (-79.5487, -28.5) ccw projected
  arc A22 (-39.3786, -106.7966) -> (-39.0027, -104.4014) centre (-40.0634, -105.462) ccw projected
  line L10 (-39.0027, -104.4014) -> (-68.324, -75.0801) projected
  line L11 (-32.9687, -39.7247) -> (-3.6474, -69.046) projected
  arc A23 (-3.6474, -69.046) -> (-1.2521, -68.6701) centre (-2.5867, -67.9854) ccw projected
  arc A24 (-1.2521, -68.6701) -> (4.2199, -55.4595) centre (-79.5487, -28.5) ccw projected
  arc A25 (4.2199, -55.4595) -> (2.792, -53.5) centre (2.792, -55) ccw projected
  line L12 (2.792, -53.5) -> (-6.0487, -53.5) projected
  arc A26 (-8.0487, -51.5) -> (-6.0487, -53.5) centre (-6.0487, -51.5) ccw projected
  line L13 (-8.0487, -51.5) -> (-8.0487, -5.5) projected
  line L14 (-94.0487, -79.9174) -> (-94.0487, -93) projected
  line L15 (-15.0487, -14) -> (-28.1313, -14) projected
  arc A27 (-30.0357, -12.6111) -> (-28.1313, -14) centre (-28.1313, -12) ccw projected
  arc A28 (-30.0357, -12.6111) -> (-63.6598, 21.0131) centre (-79.5487, -28.5) ccw projected
  arc A29 (-65.0487, 22.9174) -> (-63.6598, 21.0131) centre (-63.0487, 22.9174) ccw projected
  line L16 (-144.0487, -43) -> (-130.9661, -43) projected
  arc A30 (-129.0618, -44.3889) -> (-130.9661, -43) centre (-130.9661, -45) ccw projected
  arc A31 (-129.0618, -44.3889) -> (-95.4376, -78.0131) centre (-79.5487, -28.5) ccw projected
  arc A32 (-94.0487, -79.9174) -> (-95.4376, -78.0131) centre (-96.0487, -79.9174) ccw projected
  arc A33 (-96.0487, -95) -> (-94.0487, -93) centre (-96.0487, -93) ccw projected
  line L17 (-96.0487, -95) -> (-105.7028, -95) projected
  arc A34 (-105.7028, -95) -> (-107.2443, -95.7258) centre (-105.7028, -97) ccw projected
  line L18 (-107.2443, -95.7258) -> (-113.0806, -102.7869) projected
  arc A35 (-115.4882, -103.3155) -> (-113.0806, -102.7869) centre (-114.6222, -101.5127) ccw projected
  arc A36 (-154.3642, -64.4395) -> (-115.4882, -103.3155) centre (-79.5487, -28.5) ccw projected
  arc A37 (-153.8356, -62.0319) -> (-154.3642, -64.4395) centre (-152.5614, -63.5735) ccw projected
  line L19 (-153.8356, -62.0319) -> (-146.7745, -56.1956) projected
  arc A38 (-146.7745, -56.1956) -> (-146.0487, -54.654) centre (-148.0487, -54.654) ccw projected
  line L20 (-146.0487, -54.654) -> (-146.0487, -45) projected
  arc A39 (-144.0487, -43) -> (-146.0487, -45) centre (-144.0487, -45) ccw projected
  line L21 (-51.8531, 38.7258) -> (-46.0168, 45.7869) projected
  arc A40 (-43.6092, 46.3155) -> (-46.0168, 45.7869) centre (-44.4752, 44.5127) ccw projected
  arc A41 (-4.7333, 7.4395) -> (-43.6092, 46.3155) centre (-79.5487, -28.5) ccw projected
  arc A42 (-5.2619, 5.0319) -> (-4.7333, 7.4395) centre (-6.5361, 6.5735) ccw projected
  line L22 (-5.2619, 5.0319) -> (-12.3229, -0.8044) projected
  arc A43 (-12.3229, -0.8044) -> (-13.0487, -2.346) centre (-11.0487, -2.346) ccw projected
  line L23 (-13.0487, -2.346) -> (-13.0487, -12) projected
  arc A44 (-15.0487, -14) -> (-13.0487, -12) centre (-15.0487, -12) ccw projected
  line L24 (-65.0487, 22.9174) -> (-65.0487, 36) projected
  arc A45 (-63.0487, 38) -> (-65.0487, 36) centre (-63.0487, 36) ccw projected
  line L25 (-63.0487, 38) -> (-53.3947, 38) projected
  arc A46 (-53.3947, 38) -> (-51.8531, 38.7258) centre (-53.3947, 40) ccw projected
  arc A47 (-6.0487, -3.5) -> (-8.0487, -5.5) centre (-6.0487, -5.5) ccw projected
  line L26 (-6.0487, -3.5) -> (2.792, -3.5) projected
  arc A48 (2.792, -3.5) -> (4.2199, -1.5405) centre (2.792, -2) ccw projected
  arc A49 (4.2199, -1.5405) -> (-52.5892, 55.2686) centre (-79.5487, -28.5) ccw projected
  arc A50 (-52.5892, 55.2686) -> (-54.5487, 53.8408) centre (-53.0487, 53.8408) ccw projected
  line L27 (-54.5487, 53.8408) -> (-54.5487, 45) projected
  arc A51 (-56.5487, 43) -> (-54.5487, 45) centre (-56.5487, 45) ccw projected
  arc A52 (-153.0487, -53.5) -> (-151.0487, -51.5) centre (-153.0487, -51.5) ccw projected
  line L28 (-153.0487, -53.5) -> (-161.8895, -53.5) projected
  arc A53 (-161.8895, -53.5) -> (-163.3174, -55.4595) centre (-161.8895, -55) ccw projected
  arc A54 (-163.3174, -55.4595) -> (-106.5083, -112.2686) centre (-79.5487, -28.5) ccw projected
  arc A55 (-106.5083, -112.2686) -> (-104.5487, -110.8408) centre (-106.0487, -110.8408) ccw projected
  line L29 (-104.5487, -110.8408) -> (-104.5487, -102) projected
  arc A56 (-102.5487, -100) -> (-104.5487, -102) centre (-102.5487, -102) ccw projected
  line L30 (-90.7735, 18.0801) -> (-126.1288, -17.2753) projected
  line L31 (-68.324, -75.0801) -> (-32.9687, -39.7247) projected
  point P0 (0, 0)
  point P1 (-79.5487, -28.5)
  dimension "d46" = 98
  dimension "d47" = 2.2
  dimension "d49" = 30
  constraints: 4 end point, 3 centre point, 2 midpoint, 2 point on circle, 1 coincident, 1 equal radius
  measures "d46" diameter of A8
  measures "d47" diameter of A9
  measures "d49" angle of L0 L1
extrude "押し出し7" cut sketch "ハンドル" against normal up to surface (3 mm away) contours A9 | A10
sketch "スケッチ10" plane through (0, 0, -2) normal (0, 0, -1) x (-1, 0, 0)
  circle A0 centre (32.2184, -15.8179) radius 1.1 projected
  circle A1 centre (126.8791, -41.1821) radius 1.1 projected
  arc A2 (130.9661, -43) -> (129.0618, -44.3889) centre (130.9661, -45) ccw projected
  line L0 (130.9661, -43) -> (144.0487, -43) projected
  arc A3 (146.0487, -45) -> (144.0487, -43) centre (144.0487, -45) ccw projected
  line L1 (146.0487, -45) -> (146.0487, -54.654) projected
  arc A4 (146.0487, -54.654) -> (146.7745, -56.1956) centre (148.0487, -54.654) ccw projected
  line L2 (146.7745, -56.1956) -> (153.8356, -62.0319) projected
  arc A5 (154.3642, -64.4395) -> (153.8356, -62.0319) centre (152.5614, -63.5735) ccw projected
  arc A6 (115.4882, -103.3155) -> (154.3642, -64.4395) centre (79.5487, -28.5) ccw projected
  arc A7 (113.0806, -102.7869) -> (115.4882, -103.3155) centre (114.6222, -101.5127) ccw projected
  line L3 (113.0806, -102.7869) -> (107.2443, -95.7258) projected
  arc A8 (107.2443, -95.7258) -> (105.7028, -95) centre (105.7028, -97) ccw projected
  line L4 (105.7028, -95) -> (96.0487, -95) projected
  arc A9 (94.0487, -93) -> (96.0487, -95) centre (96.0487, -93) ccw projected
  line L5 (94.0487, -93) -> (94.0487, -79.9174) projected
  arc A10 (95.4376, -78.0131) -> (94.0487, -79.9174) centre (96.0487, -79.9174) ccw projected
  arc A11 (95.4376, -78.0131) -> (129.0618, -44.3889) centre (79.5487, -28.5) ccw projected
  line L6 (46.0168, 45.7869) -> (51.8531, 38.7258) projected
  arc A12 (51.8531, 38.7258) -> (53.3947, 38) centre (53.3947, 40) ccw projected
  line L7 (53.3947, 38) -> (63.0487, 38) projected
  arc A13 (65.0487, 36) -> (63.0487, 38) centre (63.0487, 36) ccw projected
  line L8 (65.0487, 36) -> (65.0487, 22.9174) projected
  arc A14 (63.6598, 21.0131) -> (65.0487, 22.9174) centre (63.0487, 22.9174) ccw projected
  arc A15 (63.6598, 21.0131) -> (30.0357, -12.6111) centre (79.5487, -28.5) ccw projected
  arc A16 (28.1313, -14) -> (30.0357, -12.6111) centre (28.1313, -12) ccw projected
  line L9 (28.1313, -14) -> (15.0487, -14) projected
  arc A17 (13.0487, -12) -> (15.0487, -14) centre (15.0487, -12) ccw projected
  line L10 (13.0487, -12) -> (13.0487, -2.346) projected
  arc A18 (13.0487, -2.346) -> (12.3229, -0.8044) centre (11.0487, -2.346) ccw projected
  line L11 (12.3229, -0.8044) -> (5.2619, 5.0319) projected
  arc A19 (4.7333, 7.4395) -> (5.2619, 5.0319) centre (6.5361, 6.5735) ccw projected
  arc A20 (43.6092, 46.3155) -> (4.7333, 7.4395) centre (79.5487, -28.5) ccw projected
  arc A21 (46.0168, 45.7869) -> (43.6092, 46.3155) centre (44.4752, 44.5127) ccw projected
  circle A22 centre (118.4396, -24.9645) radius 1.1 projected
  circle A23 centre (40.6579, -32.0355) radius 1.1 projected
  circle A24 centre (76.0132, -67.3909) radius 1.1 projected
  circle A25 centre (83.0843, 10.3909) radius 1.1 projected
  circle A26 centre (89.0947, -67.7444) radius 1.1 projected
  circle A27 centre (118.7932, -38.0459) radius 1.1 projected
  circle A28 centre (40.3043, -18.9541) radius 1.1 projected
  circle A29 centre (70.0028, 10.7444) radius 1.1 projected
  arc A30 (52.5892, 55.2686) -> (-4.2199, -1.5405) centre (79.5487, -28.5) ccw projected
  arc A31 (-4.2199, -1.5405) -> (-2.792, -3.5) centre (-2.792, -2) ccw projected
  line L12 (-2.792, -3.5) -> (6.0487, -3.5) projected
  arc A32 (8.0487, -5.5) -> (6.0487, -3.5) centre (6.0487, -5.5) ccw projected
  line L13 (8.0487, -5.5) -> (8.0487, -51.5) projected
  arc A33 (6.0487, -53.5) -> (8.0487, -51.5) centre (6.0487, -51.5) ccw projected
  line L14 (6.0487, -53.5) -> (-2.792, -53.5) projected
  arc A34 (-2.792, -53.5) -> (-4.2199, -55.4595) centre (-2.792, -55) ccw projected
  arc A35 (-4.2199, -55.4595) -> (1.2521, -68.6701) centre (79.5487, -28.5) ccw projected
  arc A36 (1.2521, -68.6701) -> (3.6474, -69.046) centre (2.5867, -67.9854) ccw projected
  line L15 (3.6474, -69.046) -> (32.9687, -39.7247) projected
  line L16 (32.9687, -39.7247) -> (68.324, -75.0801) projected
  line L17 (68.324, -75.0801) -> (39.0027, -104.4014) projected
  arc A37 (39.0027, -104.4014) -> (39.3786, -106.7966) centre (40.0634, -105.462) ccw projected
  arc A38 (39.3786, -106.7966) -> (52.5892, -112.2686) centre (79.5487, -28.5) ccw projected
  arc A39 (52.5892, -112.2686) -> (54.5487, -110.8408) centre (53.0487, -110.8408) ccw projected
  line L18 (54.5487, -110.8408) -> (54.5487, -102) projected
  arc A40 (56.5487, -100) -> (54.5487, -102) centre (56.5487, -102) ccw projected
  line L19 (56.5487, -100) -> (102.5487, -100) projected
  arc A41 (104.5487, -102) -> (102.5487, -100) centre (102.5487, -102) ccw projected
  line L20 (104.5487, -102) -> (104.5487, -110.8408) projected
  arc A42 (104.5487, -110.8408) -> (106.5083, -112.2686) centre (106.0487, -110.8408) ccw projected
  arc A43 (106.5083, -112.2686) -> (163.3174, -55.4595) centre (79.5487, -28.5) ccw projected
  arc A44 (163.3174, -55.4595) -> (161.8895, -53.5) centre (161.8895, -55) ccw projected
  line L21 (161.8895, -53.5) -> (153.0487, -53.5) projected
  arc A45 (151.0487, -51.5) -> (153.0487, -53.5) centre (153.0487, -51.5) ccw projected
  line L22 (151.0487, -51.5) -> (151.0487, -5.5) projected
  arc A46 (153.0487, -3.5) -> (151.0487, -5.5) centre (153.0487, -5.5) ccw projected
  line L23 (153.0487, -3.5) -> (161.8895, -3.5) projected
  arc A47 (161.8895, -3.5) -> (163.3174, -1.5405) centre (161.8895, -2) ccw projected
  arc A48 (163.3174, -1.5405) -> (157.8454, 11.6701) centre (79.5487, -28.5) ccw projected
  arc A49 (157.8454, 11.6701) -> (155.4501, 12.046) centre (156.5108, 10.9854) ccw projected
  line L24 (155.4501, 12.046) -> (126.1288, -17.2753) projected
  line L25 (126.1288, -17.2753) -> (90.7735, 18.0801) projected
  line L26 (90.7735, 18.0801) -> (120.0948, 47.4014) projected
  arc A50 (120.0948, 47.4014) -> (119.7188, 49.7966) centre (119.0341, 48.462) ccw projected
  arc A51 (119.7188, 49.7966) -> (106.5083, 55.2686) centre (79.5487, -28.5) ccw projected
  arc A52 (106.5083, 55.2686) -> (104.5487, 53.8408) centre (106.0487, 53.8408) ccw projected
  line L27 (104.5487, 53.8408) -> (104.5487, 45) projected
  arc A53 (102.5487, 43) -> (104.5487, 45) centre (102.5487, 45) ccw projected
  line L28 (102.5487, 43) -> (56.5487, 43) projected
  arc A54 (54.5487, 45) -> (56.5487, 43) centre (56.5487, 45) ccw projected
  line L29 (54.5487, 45) -> (54.5487, 53.8408) projected
  arc A55 (54.5487, 53.8408) -> (52.5892, 55.2686) centre (53.0487, 53.8408) ccw projected
  circle A56 centre (108.0487, -108.0487) radius 1.3 projected
  circle A57 centre (71.0487, 39.5) radius 0.8 projected
  circle A58 centre (88.0487, 39.5) radius 0.8 projected
  circle A59 centre (51.0487, 51.0487) radius 1.3 projected
  circle A60 centre (147.5487, -37) radius 0.8 projected
  circle A61 centre (147.5487, -20) radius 0.8 projected
  circle A62 centre (159.0975, -57) radius 1.3 projected
  circle A63 centre (71.0487, -96.5) radius 0.8 projected
  circle A64 centre (88.0487, -96.5) radius 0.8 projected
  circle A65 centre (11.5487, -37) radius 0.8 projected
  circle A66 centre (11.5487, -20) radius 0.8 projected
  circle A67 centre (0, 0) radius 1.3 projected
  line L30 (63.6598, 21.0131) -> (30.0357, -12.6111)
  line L31 (129.0618, -44.3889) -> (95.4376, -78.0131)
  line L32 (18.8265, -53.8669) -> (54.1819, -89.2222)
  line L33 (68.324, -75.0801) -> (32.9687, -39.7247) projected
  line L34 (104.9156, 32.2222) -> (140.2709, -3.1331)
  line L35 (90.7735, 18.0801) -> (126.1288, -17.2753) projected
  point P0 (0, 0)
  dimension "d85" = 20
  dimension "d86" = 20
  constraints: 8 end point, 4 point on line, 3 parallel, 1 perpendicular
  measures "d85" distance between parallel lines of L32 L33
  measures "d86" distance between parallel lines of L25 L34
extrude "押し出し10" cut sketch "スケッチ10" against normal up to surface (3 mm away) contours A11 L31 | L30 A15
extrude "押し出し11" add sketch "スケッチ10" against normal up to surface (3 mm away) contours L34 L24 L25 L26 | L15 L16 L17 L32
fillet "フィレット3" radius 2 4 edges at (-104.9156, 32.2222, -0.5) (-140.2709, -3.1331, -0.5) (-18.8265, -53.8669, -0.5) (-54.1819, -89.2222, -0.5)